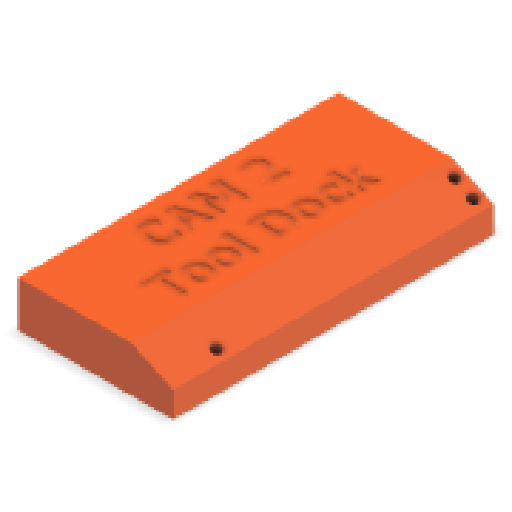
# Autodesk Inventor part: Waveshare Cam Holder - Tool Dock
Saved by Autodesk Inventor 2023.2 (Build 272271000, 271)
## iProperties
Created: 2023-02-26
Part Number: Waveshare Cam Holder - Tool Dock
Material: ABS Plastic
Document SubType Name: Modeling
Designer: remop
Density: 1.06 g/cm^3
Appearance: Smooth - Light Orange
Author: remop
Autodesk Inventor part; units mm, degrees
ref_plane "YZ Plane" through (0, 0, 0) normal (1, 0, 0) x (0, 1, 0)
ref_plane "XZ Plane" through (0, 0, 0) normal (0, 1, 0) x (-1, 0, 0)
ref_plane "XY Plane" through (0, 0, 0) normal (0, 0, 1) x (1, 0, 0)
sketch "Sketch1" plane through (0, 0, 0) normal (0, 0, 1) x (1, 0, 0)
  line L0 (0, 0) -> (0, 5)
  line L1 (0, 5) -> (-8.1568, 8.8036)
  line L2 (-8.1568, 8.8036) -> (-30, 8.8036)
  line L3 (-30, 8.8036) -> (-30, 0)
  line L4 (-30, 0) -> (0, 0)
  dimension "d0" = 65
  dimension "d1" = 5
  dimension "d2" = 30
  dimension "d3" = 9
  constraints: 10 end point, 3 perpendicular, 1 vertical
  measures "d0" angle of L0 L1
  measures "d1" distance of L0.start L0.end
  measures "d2" distance of L3.end L0.start
  measures "d3" distance of L0.end L1.end
extrude "Extrusion1" add sketch "Sketch1" along normal blind 62
sketch "Sketch2" plane through (-8.1568, 8.8036, 62) normal (0.4226183, 0.9063078, 0) x (0.9063078, -0.4226183, 0)
  line L0 (9, 62) -> (0, 62) projected
  line L1 (0, 62) -> (0, 0) projected
  line L2 (9, 0) -> (0, 0) projected
  line L3 (9, 62) -> (9, 0) projected
  point P0 (11.1131, 62)
  point P1 (2.75, 60)
  point P2 (6.75, 60)
  point P3 (7, 10.2)
  dimension "d6" = 2
  dimension "d7" = 2.75
  dimension "d8" = 4
  dimension "d9" = 2
  dimension "d10" = 49.8
  constraints: 1 horizontal alignment
  measures "d6" distance from line of L3 point (7, 10.2)
  measures "d7" distance from line of L1 point (2.75, 60)
  measures "d8" distance of point (2.75, 60) point (6.75, 60)
  measures "d9" distance from line of L0 point (6.75, 60)
  measures "d10" vertical distance of point (6.75, 60) point (7, 10.2)
hole "Hole1" at (-5.6644, 7.6414, 2) at (-2.0392, 5.9509, 2) at (-1.8126, 5.8452, 51.8) direction (-0.4226183, -0.9063078, 0) diameter 2 end through all
sketch "Sketch3" plane through (-30, 0, 0) normal (-1, 0, 0) x (0, 0, 1)
  line L0 (0, 8.8036) -> (0, 0) projected
  line L1 (0, 0) -> (62, 0) projected
  line L2 (62, 8.8036) -> (62, 0) projected
  line L3 (0, 8.8036) -> (62, 8.8036) projected
  point P0 (0, 0)
  point P1 (6, 4.4018)
  point P2 (56, 4.4018)
  point P3 (0, 4.4018)
  point P4 (62, 4.4018)
  dimension "d18" = 62
  dimension "d19" = 6
  dimension "d20" = 6
  constraints: 2 horizontal alignment, 2 midpoint
  measures "d18" distance of L0.start L2.start
  measures "d19" distance from line of L0 point (6, 4.402)
  measures "d20" distance from line of L2 point (56, 4.402)
hole "Hole2" at (-30, 4.4018, 6) at (-30, 4.4018, 56) direction (1, 0, 0) diameter 2.9 depth 15 tip angle 118
sketch "Sketch4" plane through (-30, 8.8036, 0) normal (0, 1, 0) x (1, 0, 0)
  line L0 (21.8432, 0) -> (0, 0) projected
  line L1 (0, 0) -> (0, -62) projected
  line L2 (21.8432, -62) -> (0, -62) projected
  line L3 (21.8432, 0) -> (21.8432, -62) projected
  line L4 (0, -62) -> (0, 0) construction
  line L5 (0, 0) -> (21.8432, 0) construction
  line L6 (21.8432, 0) -> (21.8432, -62) construction
  line L7 (21.8432, -62) -> (0, -62) construction
  spline S0 degree 2 poles (9.0867, -40.8922) (9.0867, -42.2439) (7.453, -43.829) (5.9749, -43.829) knots 0 0 0 1 2 2 2
  spline S1 degree 2 poles (5.9749, -43.829) (4.5503, -43.829) (2.8533, -42.2391) (2.8533, -40.8874) knots 0 0 0 1 2 2 2
  spline S2 degree 2 poles (2.8533, -40.8874) (2.8533, -40.5324) (2.936, -39.9587) (3.0041, -39.6961) knots 0 0 0 1 2 2 2
  spline S3 degree 2 poles (3.0041, -39.6961) (3.0673, -39.4919) (3.2764, -39.0105) (3.3542, -38.8598) knots 0 0 0 1 2 2 2
  line L8 (3.3542, -38.8598) -> (4.7837, -38.8598)
  line L9 (4.7837, -38.8598) -> (4.7837, -39.0105)
  spline S4 degree 2 poles (4.7837, -39.0105) (4.6864, -39.1224) (4.4141, -39.453) (4.2877, -39.6621) knots 0 0 0 1 2 2 2
  spline S5 degree 2 poles (4.2877, -39.6621) (4.1564, -39.8712) (3.9765, -40.372) (3.9765, -40.6491) knots 0 0 0 1 2 2 2
  spline S6 degree 2 poles (3.9765, -40.6491) (3.9765, -40.9749) (4.1807, -41.5146) (4.4384, -41.7626) knots 0 0 0 1 2 2 2
  spline S7 degree 2 poles (4.4384, -41.7626) (4.667, -41.9862) (5.4498, -42.2731) (5.9798, -42.2731) knots 0 0 0 1 2 2 2
  spline S8 degree 2 poles (5.9798, -42.2731) (6.5389, -42.2731) (7.3023, -41.9765) (7.5357, -41.7334) knots 0 0 0 1 2 2 2
  spline S9 degree 2 poles (7.5357, -41.7334) (7.7642, -41.5) (7.9636, -40.9263) (7.9636, -40.6394) knots 0 0 0 1 2 2 2
  spline S10 degree 2 poles (7.9636, -40.6394) (7.9636, -40.3428) (7.7642, -39.8031) (7.6426, -39.6183) knots 0 0 0 1 2 2 2
  spline S11 degree 2 poles (7.6426, -39.6183) (7.5211, -39.4141) (7.2634, -39.1078) (7.1613, -38.9959) knots 0 0 0 1 2 2 2
  line L10 (7.1613, -38.9959) -> (7.1613, -38.8598)
  line L11 (7.1613, -38.8598) -> (8.5713, -38.8598)
  spline S12 degree 2 poles (8.5713, -38.8598) (8.6491, -39.0251) (8.8436, -39.4579) (8.9117, -39.6912) knots 0 0 0 1 2 2 2
  spline S13 degree 2 poles (8.9117, -39.6912) (8.9992, -39.9733) (9.0867, -40.4643) (9.0867, -40.8922) knots 0 0 0 1 2 2 2
  line L12 (8.97, -38.6167) -> (2.97, -36.5891)
  line L13 (2.97, -36.5891) -> (2.97, -34.9457)
  line L14 (2.97, -34.9457) -> (8.97, -32.9182)
  line L15 (8.97, -32.9182) -> (8.97, -34.4692)
  line L16 (8.97, -34.4692) -> (7.7448, -34.8436)
  line L17 (7.7448, -34.8436) -> (7.7448, -36.7301)
  line L18 (7.7448, -36.7301) -> (8.97, -37.1094)
  line L19 (8.97, -37.1094) -> (8.97, -38.6167)
  line L20 (6.6556, -35.1742) -> (4.6718, -35.7869)
  line L21 (4.6718, -35.7869) -> (6.6556, -36.4044)
  line L22 (6.6556, -36.4044) -> (6.6556, -35.1742)
  line L23 (8.97, -26.1937) -> (8.97, -27.6912)
  line L24 (8.97, -27.6912) -> (4.9927, -27.6912)
  line L25 (4.9927, -27.6912) -> (7.56, -28.7804)
  line L26 (7.56, -28.7804) -> (7.56, -29.8112)
  line L27 (7.56, -29.8112) -> (4.9927, -30.9003)
  line L28 (4.9927, -30.9003) -> (8.97, -30.9003)
  line L29 (8.97, -30.9003) -> (8.97, -32.3201)
  line L30 (8.97, -32.3201) -> (2.97, -32.3201)
  line L31 (2.97, -32.3201) -> (2.97, -30.5843)
  line L32 (2.97, -30.5843) -> (5.9311, -29.252)
  line L33 (5.9311, -29.252) -> (2.97, -27.9295)
  line L34 (2.97, -27.9295) -> (2.97, -26.1937)
  line L35 (2.97, -26.1937) -> (8.97, -26.1937)
  line L36 (8.97, -18.137) -> (8.97, -22.547)
  line L37 (8.97, -22.547) -> (7.9927, -22.547)
  spline S14 degree 2 poles (7.9927, -22.547) (7.5454, -21.9878) (6.7577, -21.0932) (6.4028, -20.7577) knots 0 0 0 1 2 2 2
  spline S15 degree 2 poles (6.4028, -20.7577) (5.9409, -20.3152) (5.2358, -19.9214) (4.8663, -19.9214) knots 0 0 0 1 2 2 2
  spline S16 degree 2 poles (4.8663, -19.9214) (4.4482, -19.9214) (4.0008, -20.4222) (4.0008, -20.8695) knots 0 0 0 1 2 2 2
  spline S17 degree 2 poles (4.0008, -20.8695) (4.0008, -21.0981) (4.1127, -21.5065) (4.2002, -21.7156) knots 0 0 0 1 2 2 2
  spline S18 degree 2 poles (4.2002, -21.7156) (4.2926, -21.9198) (4.4871, -22.2115) (4.5357, -22.2844) knots 0 0 0 1 2 2 2
  line L38 (4.5357, -22.2844) -> (4.5357, -22.4011)
  line L39 (4.5357, -22.4011) -> (3.2277, -22.4011)
  spline S19 degree 2 poles (3.2277, -22.4011) (3.1062, -22.1483) (2.8533, -21.0689) (2.8533, -20.5681) knots 0 0 0 1 2 2 2
  spline S20 degree 2 poles (2.8533, -20.5681) (2.8533, -19.4984) (3.8063, -18.3995) (4.667, -18.3995) knots 0 0 0 1 2 2 2
  spline S21 degree 2 poles (4.667, -18.3995) (5.1969, -18.3995) (6.218, -18.9003) (6.8015, -19.4789) knots 0 0 0 1 2 2 2
  spline S22 degree 2 poles (6.8015, -19.4789) (7.1613, -19.8436) (7.7204, -20.5292) (7.8371, -20.6799) knots 0 0 0 1 2 2 2
  line L40 (7.8371, -20.6799) -> (7.8371, -18.137)
  line L41 (7.8371, -18.137) -> (8.97, -18.137)
  line L42 (18.8489, -49.6272) -> (13.9915, -49.6272)
  line L43 (13.9915, -49.6272) -> (13.9915, -51.4019)
  line L44 (13.9915, -51.4019) -> (12.8489, -51.4019)
  line L45 (12.8489, -51.4019) -> (12.8489, -46.3452)
  line L46 (12.8489, -46.3452) -> (13.9915, -46.3452)
  line L47 (13.9915, -46.3452) -> (13.9915, -48.1199)
  line L48 (13.9915, -48.1199) -> (18.8489, -48.1199)
  line L49 (18.8489, -48.1199) -> (18.8489, -49.6272)
  spline S23 degree 2 poles (16.5879, -41.4684) (17.7063, -41.4684) (18.9899, -42.6888) (18.9899, -43.8023) knots 0 0 0 1 2 2 2
  spline S24 degree 2 poles (18.9899, -43.8023) (18.9899, -44.9109) (17.7063, -46.141) (16.5879, -46.141) knots 0 0 0 1 2 2 2
  spline S25 degree 2 poles (16.5879, -46.141) (15.4599, -46.141) (14.1811, -44.9109) (14.1811, -43.8023) knots 0 0 0 1 2 2 2
  spline S26 degree 2 poles (14.1811, -43.8023) (14.1811, -42.6937) (15.4648, -41.4684) (16.5879, -41.4684) knots 0 0 0 1 2 2 2
  spline S27 degree 2 poles (16.5977, -42.9125) (16.1941, -42.9125) (15.6544, -43.0438) (15.4939, -43.1605) knots 0 0 0 1 2 2 2
  spline S28 degree 2 poles (15.4939, -43.1605) (15.3238, -43.2869) (15.1925, -43.6029) (15.1925, -43.8023) knots 0 0 0 1 2 2 2
  spline S29 degree 2 poles (15.1925, -43.8023) (15.1925, -43.9968) (15.3092, -44.3031) (15.4745, -44.4295) knots 0 0 0 1 2 2 2
  spline S30 degree 2 poles (15.4745, -44.4295) (15.6301, -44.5511) (16.1795, -44.6969) (16.5977, -44.6969) knots 0 0 0 1 2 2 2
  spline S31 degree 2 poles (16.5977, -44.6969) (17.011, -44.6969) (17.5215, -44.5608) (17.6771, -44.4489) knots 0 0 0 1 2 2 2
  spline S32 degree 2 poles (17.6771, -44.4489) (17.8327, -44.3371) (17.9785, -43.9968) (17.9785, -43.7925) knots 0 0 0 1 2 2 2
  spline S33 degree 2 poles (17.9785, -43.7925) (17.9785, -43.6224) (17.8327, -43.2723) (17.6868, -43.1653) knots 0 0 0 1 2 2 2
  spline S34 degree 2 poles (17.6868, -43.1653) (17.5166, -43.0438) (17.0255, -42.9125) (16.5977, -42.9125) knots 0 0 0 1 2 2 2
  spline S35 degree 2 poles (16.5879, -36.3776) (17.7063, -36.3776) (18.9899, -37.5981) (18.9899, -38.7115) knots 0 0 0 1 2 2 2
  spline S36 degree 2 poles (18.9899, -38.7115) (18.9899, -39.8201) (17.7063, -41.0502) (16.5879, -41.0502) knots 0 0 0 1 2 2 2
  spline S37 degree 2 poles (16.5879, -41.0502) (15.4599, -41.0502) (14.1811, -39.8201) (14.1811, -38.7115) knots 0 0 0 1 2 2 2
  spline S38 degree 2 poles (14.1811, -38.7115) (14.1811, -37.6029) (15.4648, -36.3776) (16.5879, -36.3776) knots 0 0 0 1 2 2 2
  spline S39 degree 2 poles (16.5977, -37.8217) (16.1941, -37.8217) (15.6544, -37.953) (15.4939, -38.0697) knots 0 0 0 1 2 2 2
  spline S40 degree 2 poles (15.4939, -38.0697) (15.3238, -38.1961) (15.1925, -38.5122) (15.1925, -38.7115) knots 0 0 0 1 2 2 2
  spline S41 degree 2 poles (15.1925, -38.7115) (15.1925, -38.906) (15.3092, -39.2123) (15.4745, -39.3387) knots 0 0 0 1 2 2 2
  spline S42 degree 2 poles (15.4745, -39.3387) (15.6301, -39.4603) (16.1795, -39.6062) (16.5977, -39.6062) knots 0 0 0 1 2 2 2
  spline S43 degree 2 poles (16.5977, -39.6062) (17.011, -39.6062) (17.5215, -39.47) (17.6771, -39.3582) knots 0 0 0 1 2 2 2
  spline S44 degree 2 poles (17.6771, -39.3582) (17.8327, -39.2464) (17.9785, -38.906) (17.9785, -38.7018) knots 0 0 0 1 2 2 2
  spline S45 degree 2 poles (17.9785, -38.7018) (17.9785, -38.5316) (17.8327, -38.1815) (17.6868, -38.0746) knots 0 0 0 1 2 2 2
  spline S46 degree 2 poles (17.6868, -38.0746) (17.5166, -37.953) (17.0255, -37.8217) (16.5977, -37.8217) knots 0 0 0 1 2 2 2
  line L50 (18.8489, -34.2188) -> (18.8489, -35.6288)
  line L51 (18.8489, -35.6288) -> (12.5815, -35.6288)
  line L52 (12.5815, -35.6288) -> (12.5815, -34.2188)
  line L53 (12.5815, -34.2188) -> (18.8489, -34.2188)
  spline S47 degree 2 poles (15.8537, -25.2869) (16.6949, -25.2869) (18.0174, -26.0211) (18.3724, -26.5802) knots 0 0 0 1 2 2 2
  spline S48 degree 2 poles (18.3724, -26.5802) (18.6738, -27.047) (18.8489, -28.1459) (18.8489, -28.7634) knots 0 0 0 1 2 2 2
  line L54 (18.8489, -28.7634) -> (18.8489, -30.6402)
  line L55 (18.8489, -30.6402) -> (12.8489, -30.6402)
  line L56 (12.8489, -30.6402) -> (12.8489, -28.7828)
  spline S49 degree 2 poles (12.8489, -28.7828) (12.8489, -28.1507) (13.0093, -27.047) (13.3205, -26.5608) knots 0 0 0 1 2 2 2
  spline S50 degree 2 poles (13.3205, -26.5608) (13.6998, -25.9724) (14.9834, -25.2869) (15.8537, -25.2869) knots 0 0 0 1 2 2 2
  spline S51 degree 2 poles (15.844, -26.8331) (15.2508, -26.8331) (14.4048, -27.2415) (14.1665, -27.6596) knots 0 0 0 1 2 2 2
  spline S52 degree 2 poles (14.1665, -27.6596) (14.0012, -27.966) (13.9672, -28.637) (13.9672, -29.1037) knots 0 0 0 1 2 2 2
  line L57 (13.9672, -29.1037) -> (13.9672, -29.1329)
  line L58 (13.9672, -29.1329) -> (17.7257, -29.1329)
  line L59 (17.7257, -29.1329) -> (17.7257, -29.1037)
  spline S53 degree 2 poles (17.7257, -29.1037) (17.7257, -28.5981) (17.6917, -27.9028) (17.4923, -27.5867) knots 0 0 0 1 2 2 2
  spline S54 degree 2 poles (17.4923, -27.5867) (17.2589, -27.2172) (16.4372, -26.8331) (15.844, -26.8331) knots 0 0 0 1 2 2 2
  spline S55 degree 2 poles (16.5879, -20.1329) (17.7063, -20.1329) (18.9899, -21.3533) (18.9899, -22.4668) knots 0 0 0 1 2 2 2
  spline S56 degree 2 poles (18.9899, -22.4668) (18.9899, -23.5754) (17.7063, -24.8055) (16.5879, -24.8055) knots 0 0 0 1 2 2 2
  spline S57 degree 2 poles (16.5879, -24.8055) (15.4599, -24.8055) (14.1811, -23.5754) (14.1811, -22.4668) knots 0 0 0 1 2 2 2
  spline S58 degree 2 poles (14.1811, -22.4668) (14.1811, -21.3582) (15.4648, -20.1329) (16.5879, -20.1329) knots 0 0 0 1 2 2 2
  spline S59 degree 2 poles (16.5977, -21.577) (16.1941, -21.577) (15.6544, -21.7083) (15.4939, -21.825) knots 0 0 0 1 2 2 2
  spline S60 degree 2 poles (15.4939, -21.825) (15.3238, -21.9514) (15.1925, -22.2674) (15.1925, -22.4668) knots 0 0 0 1 2 2 2
  spline S61 degree 2 poles (15.1925, -22.4668) (15.1925, -22.6613) (15.3092, -22.9676) (15.4745, -23.094) knots 0 0 0 1 2 2 2
  spline S62 degree 2 poles (15.4745, -23.094) (15.6301, -23.2156) (16.1795, -23.3614) (16.5977, -23.3614) knots 0 0 0 1 2 2 2
  spline S63 degree 2 poles (16.5977, -23.3614) (17.011, -23.3614) (17.5215, -23.2253) (17.6771, -23.1135) knots 0 0 0 1 2 2 2
  spline S64 degree 2 poles (17.6771, -23.1135) (17.8327, -23.0016) (17.9785, -22.6613) (17.9785, -22.457) knots 0 0 0 1 2 2 2
  spline S65 degree 2 poles (17.9785, -22.457) (17.9785, -22.2869) (17.8327, -21.9368) (17.6868, -21.8298) knots 0 0 0 1 2 2 2
  spline S66 degree 2 poles (17.6868, -21.8298) (17.5166, -21.7083) (17.0255, -21.577) (16.5977, -21.577) knots 0 0 0 1 2 2 2
  spline S67 degree 2 poles (18.9704, -17.1669) (18.9704, -17.7261) (18.6884, -18.6548) (18.3967, -19) knots 0 0 0 1 2 2 2
  spline S68 degree 2 poles (18.3967, -19) (18.1001, -19.3355) (17.2103, -19.7147) (16.6074, -19.7147) knots 0 0 0 1 2 2 2
  spline S69 degree 2 poles (16.6074, -19.7147) (15.9558, -19.7147) (15.0466, -19.3063) (14.7549, -18.9514) knots 0 0 0 1 2 2 2
  spline S70 degree 2 poles (14.7549, -18.9514) (14.4729, -18.6159) (14.2006, -17.7018) (14.2006, -17.2058) knots 0 0 0 1 2 2 2
  spline S71 degree 2 poles (14.2006, -17.2058) (14.2006, -16.8314) (14.3756, -16.0827) (14.5653, -15.7034) knots 0 0 0 1 2 2 2
  line L60 (14.5653, -15.7034) -> (15.7711, -15.7034)
  line L61 (15.7711, -15.7034) -> (15.7711, -15.8833)
  spline S72 degree 2 poles (15.7711, -15.8833) (15.6884, -15.9708) (15.4939, -16.2139) (15.4161, -16.3598) knots 0 0 0 1 2 2 2
  spline S73 degree 2 poles (15.4161, -16.3598) (15.3286, -16.5154) (15.2119, -16.8995) (15.2119, -17.1378) knots 0 0 0 1 2 2 2
  spline S74 degree 2 poles (15.2119, -17.1378) (15.2119, -17.6775) (15.9656, -18.2707) (16.6074, -18.2707) knots 0 0 0 1 2 2 2
  spline S75 degree 2 poles (16.6074, -18.2707) (17.2881, -18.2707) (17.9591, -17.6386) (17.9591, -17.1135) knots 0 0 0 1 2 2 2
  spline S76 degree 2 poles (17.9591, -17.1135) (17.9591, -16.846) (17.8375, -16.4473) (17.75, -16.3015) knots 0 0 0 1 2 2 2
  spline S77 degree 2 poles (17.75, -16.3015) (17.6674, -16.1605) (17.4826, -15.9562) (17.4097, -15.8833) knots 0 0 0 1 2 2 2
  line L62 (17.4097, -15.8833) -> (17.4097, -15.7034)
  line L63 (17.4097, -15.7034) -> (18.6204, -15.7034)
  spline S78 degree 2 poles (18.6204, -15.7034) (18.6738, -15.825) (18.81, -16.141) (18.8537, -16.3063) knots 0 0 0 1 2 2 2
  spline S79 degree 2 poles (18.8537, -16.3063) (18.9121, -16.5105) (18.9704, -16.8703) (18.9704, -17.1669) knots 0 0 0 1 2 2 2
  line L64 (18.8489, -10.5008) -> (18.8489, -12.1783)
  line L65 (18.8489, -12.1783) -> (16.8845, -13.4036)
  line L66 (16.8845, -13.4036) -> (17.1763, -13.6224)
  line L67 (17.1763, -13.6224) -> (18.8489, -13.6224)
  line L68 (18.8489, -13.6224) -> (18.8489, -15.0324)
  line L69 (18.8489, -15.0324) -> (12.5815, -15.0324)
  line L70 (12.5815, -15.0324) -> (12.5815, -13.6224)
  line L71 (12.5815, -13.6224) -> (16.092, -13.6224)
  line L72 (16.092, -13.6224) -> (14.3221, -12.2852)
  line L73 (14.3221, -12.2852) -> (14.3221, -10.6175)
  line L74 (14.3221, -10.6175) -> (16.2719, -12.2026)
  line L75 (16.2719, -12.2026) -> (18.8489, -10.5008)
  point P0 (30, 0)
  constraints: 3 coincident, 1 vertical alignment, 2 other
extrude "Extrusion2" cut sketch "Sketch4" against normal blind 0.4 contours S0 S1 S2 S3 L8 L9 S4 S5 S6 S7 S8 S9 S10 S11 L10 L11 S12 S13 | L12 L13 L14 L15 L16 L17 L18 L19 | L23 L24 L25 L26 L27 L28 L29 L30 L31 L32 L33 L34 L35 | L36 L37 S14 S15 S16 S17 S18 L38 L39 S19 S20 S21 S22 L40 L41 | L42 L43 L44 L45 L46 L47 L48 L49 | S23 S24 S25 S26 | S35 S36 S37 S38 | L50 L51 L52 L53 | S47 S48 L54 L55 L56 S49 S50 | S55 S56 S57 S58 | S67 S68 S69 S70 S71 L60 L61 S72 S73 S74 S75 S76 S77 L62 L63 S78 S79 | L64 L65 L66 L67 L68 L69 L70 L71 L72 L73 L74 L75
equation "\"d20\" = d19"
body "Solid1"
